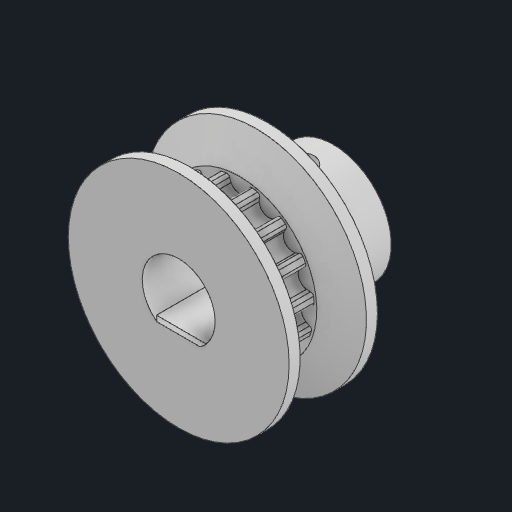
# Autodesk Inventor part: EncoderPully
Saved by Autodesk Inventor 2022.2 (Build 262287000, 287)
## iProperties
Created: 2022-11-13
Part Number: EncoderPully
Material: Generic
Document SubType Name: Modeling
Designer: haash
Density: 1 g/cm^3
Appearance: Default
Author: haash
Autodesk Inventor part; units mm, degrees
note: some values were not read from the file. Left out: dimensions or parameters whose unit could not be read.
ref_plane "YZ Plane" through (0, 0, 0) normal (1, 0, 0) x (0, 1, 0)
ref_plane "XZ Plane" through (0, 0, 0) normal (0, 1, 0) x (-1, 0, 0)
ref_plane "XY Plane" through (0, 0, 0) normal (0, 0, 1) x (1, 0, 0)
sketch "Sketch1" plane through (0, 0, 0) normal (0, 0, 1) x (1, 0, 0)
  circle A0 centre (0, 0) radius 7.162 construction
  circle A1 centre (0, 0) radius 6.781
  line L0 (0, 0) -> (0, 6.781) construction
  circle A2 centre (-0.604, 6.781) radius 1.52
  circle A3 centre (0, 6.491) radius 0.85
  circle A4 centre (-1.1313, 6.4322) radius 0.25
  circle A5 centre (0, 0) radius 6.281 construction
  circle A6 centre (0.604, 6.781) radius 1.52
  circle A7 centre (1.1313, 6.4322) radius 0.25
  point P0 (0, 5.641)
  point P1 (0, 5.641)
  point P2 (-0.7663, 6.1231)
  point P3 (-0.8862, 6.4815)
  point P4 (-1.1746, 6.6785)
  point P5 (1.1746, 6.6785)
  point P6 (0.8862, 6.4815)
  point P7 (0.7663, 6.1231)
  dimension "d9" = 13.5619
  dimension "d0" = 14.3239
  dimension "d1" = 0.381
  dimension "d2" = 0.5
  dimension "d3" = 1.7
  dimension "d5" = 3.04
  dimension "d7" = 1.14
  dimension "d8" = 12.5619
  constraints: 7 centre point, 3 coincident, 3 point on line, 3 tangent, 2 end point, 2 point on circle, 2 symmetric about line, 1 horizontal alignment, 1 vertical, 5 other
  measures "d0" diameter of A0
  measures "d2" diameter of A4
  measures "d3" diameter of A3
  measures "d5" diameter of A2
  measures "d7" distance of L0.end A3.end
  measures "d8" diameter of A5
extrude "Extrusion2" add sketch "Sketch1" along normal mid plane 3 contours A1 A2 A6 | A6 A2 A7 A1 | A1 A4 A6 A2 | A7 A2 A1 | A7 | A6 A3 A2 | A1 A6 A4 | A4 | A2 A3 A1 | A3 A1 | A6 A1 A3 picked at (-0.2976, -2.7323) picked at (-0.0353, 6.3996)
extrude "Extrusion3" cut sketch "Sketch1" along normal through all both and the other way through all contours A7 A2 A1 | A1 A6 A4 | A2 A3 A1 | A3 A1 | A6 A1 A3 picked at (-0.0353, 6.3996)
pattern_circular "Circular Pattern1" count 15 over 360 about axis through (0, 0, 0) along (0, 0, 1) of "Extrusion3"
sketch "Sketch2" plane through (0, 0, -1.5) normal (0, 0, -1) x (-1, 0, 0)
  circle A0 centre (0, 0) radius 10
  dimension "d19" = 20
  constraints: 1 centre point, 1 coincident
  measures "d19" diameter of A0
extrude "Extrusion4" add sketch "Sketch2" along normal blind 2.5
sketch "Sketch3" plane through (0, 0, 0) normal (1, 0, 0) x (0, 1, 0)
  line L0 (-10, -1.5) -> (10, -1.5) projected
  line L1 (10, -1.5) -> (10, -4) projected
  line L2 (10, -3) -> (7, -1.5)
  line L3 (0, -5.1) -> (0, 2.6) projected
  point P0 (0, 0)
  dimension "d22" = 1.5
  dimension "d23" = 3
  constraints: 2 end point, 2 point on line
  measures "d22" vertical distance of L2.start L2.end
  measures "d23" horizontal distance of L2.start L2.end
revolve "Revolution1" cut sketch "Sketch3" angle 360 about axis through (0, 0, -10) along (0, 0, 1)
mirror "Mirror1" about plane through (0, 0, 0) normal (0, 0, 1) of "Revolution1", "Extrusion4"
sketch "Sketch4" plane through (0, 0, -4) normal (0, 0, -1) x (-1, 0, 0)
  circle A0 centre (0, 0) radius 5.25
  dimension "d25" = 10.5
  constraints: 1 centre point, 1 coincident
  measures "d25" diameter of A0
extrude "Extrusion5" add sketch "Sketch4" along normal blind 6
sketch "Sketch5" plane through (0, 0, -10) normal (0, 0, -1) x (-1, 0, 0)
  circle A0 centre (0, 0) radius 3.3
  dimension "d28" = 6.6
  constraints: 1 centre point, 1 coincident
  measures "d28" diameter of A0
extrude "Extrusion6" cut sketch "Sketch5" along normal through all both and the other way through all
sketch "Sketch6" plane through (0, 0, 4) normal (0, 0, 1) x (1, 0, 0)
  circle A0 centre (0, 0) radius 3.3 projected
  line L0 (-2.265, -2.4) -> (2.265, -2.4)
  point P0 (0, -2.4)
  dimension "d31" = 2.4
  constraints: 2 end point, 2 point on circle, 1 horizontal, 1 midpoint
  measures "d31" distance of point (0, 0) point (0, -2.4)
extrude "Extrusion7" add sketch "Sketch6" against normal blind 5.25 contours L0 A0 picked at (-0.5659, -2.5433)
chamfer "Chamfer1" distance 0.25 angle 45 1 edges at (0, -2.4, 4)
sketch "Sketch7" plane through (0, 0, 0) normal (0, 1, 0) x (-1, 0, 0)
  circle A0 centre (0, -7) radius 1.25
  line L0 (-10, -4) -> (10, -4) projected
  line L1 (-5.25, -10) -> (5.25, -10) projected
  point P0 (0, 0)
  dimension "d37" = 2.5
  dimension "d38" = 3
  dimension "d39" = 3
  constraints: 1 centre point, 1 vertical alignment
  measures "d37" diameter of A0
  measures "d38" distance from line of A0.centre L0
  measures "d39" distance from line of L1 A0.centre
extrude "Extrusion8" cut sketch "Sketch7" along normal through all both and the other way through all
equation "\"d0\" = PCD"
equation "\"d1\" = PLD"
equation "\"d2\" = 2 * R1"
equation "\"d3\" = 2 * R3"
equation "\"d5\" = 2 * R2"
equation "\"d7\" = h2"
equation "\"d8\" = d9 - 2 * d2"
equation "\"d38\" = d39"
equation "\"Pitch\" = 3"
equation "\"R1\" = 0.25"
equation "\"R2\" = 1.52"
equation "\"R3\" = 0.85"
equation "\"b\" = 0.61"
equation "\"Height\" = 1.38"
equation "\"h2\" = 1.14"
equation "\"PLD\" = 0.381"
equation "\"PCD\" = 14.323945"
body "Solid2"
